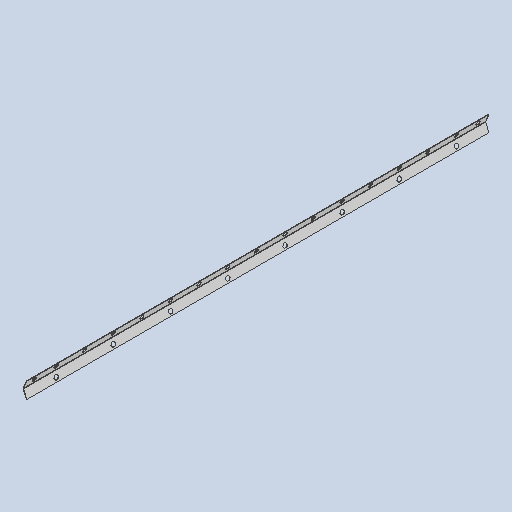
# Autodesk Inventor part: DMF 01 17 опора крышки v2.1
Saved by Autodesk Inventor 2025 (Build 290162010, 162A)
## iProperties
Created: 2024-04-30
Part Number: DMF 01 17 опора крышки v2.1
Material: Generic
Document SubType Name: Sheet Metal
Designer: pokla
Density: 1 g/cm^3
Appearance: Default
Sheet Metal Rule: Default
Flat Pattern Width: 7.47819 cm
Flat Pattern Length: 202 cm
Flat Pattern Area: 1510.6 cm^2
Sheet Metal Width: 74,782 mm
Sheet Metal Length: 2020,000 mm
Sheet Metal Area: 151059,532 mm^2
Stock Number: Барабан_Полка_Крышки
Author: pokla
Autodesk Inventor part; units mm, degrees
ref_plane "YZ Plane" through (0, 0, 0) normal (1, 0, 0) x (0, 1, 0)
ref_plane "XZ Plane" through (0, 0, 0) normal (0, 1, 0) x (-1, 0, 0)
ref_plane "XY Plane" through (0, 0, 0) normal (0, 0, 1) x (1, 0, 0)
sketch "Sketch4" plane through (0, 0, 0) normal (0, 0, 1) x (1, 0, 0)
  line L0 (-195.551234, 195.551234) -> (0, 276.551207) construction
  line L1 (0, 276.551207) -> (195.551234, 195.551234) construction
  line L2 (195.551234, 195.551234) -> (276.551207, 0) construction
  line L3 (276.551207, 0) -> (195.551234, -195.551234) construction
  line L4 (195.551234, -195.551234) -> (0, -276.551207) construction
  line L5 (0, -276.551207) -> (-195.551234, -195.551234) construction
  line L6 (-195.551234, -195.551234) -> (-276.551207, 0) construction
  line L7 (-276.551207, 0) -> (-195.551234, 195.551234) construction
  line L8 (-275.917157, 1.530734) -> (-262.041055, 35.030606)
  line L9 (-275.917157, -1.530734) -> (-262.041055, -35.030606)
  arc A0 (-275.917157, 1.530734) -> (-275.917157, -1.530734) centre (-272.221638, 0) ccw
  point P0 (0, 0)
  point P1 (0, 0)
  point P2 (0, 0)
  dimension "d16" = 511
  dimension "d23" = 36.26
  dimension "d24" = 4
  measures "d16" distance between parallel lines of L7 L3
  measures "d23" distance of L8.start L8.end
  measures "d24" radius of A0
contour flange "Contour Flange1" sketch "Sketch4" thickness 2 bend radius 2 width 2020 along (0, 0, -1) mid plane no both sides no wall seen from (-268.979106, 18.28067, 0) lies toward (0.9238795, -0.3826834, 0) curves L8 A0 L9
bend "Bend2"
corner "Corner2"
sketch "Sketch6" plane through (-275.917157, 1.530734, 0) normal (-0.9238795, 0.3826834, 0) x (0.3826834, 0.9238795, 0)
  circle A0 centre (19.22, 40.75) radius 5.5 construction
  circle A1 centre (19.22, 1979.25) radius 5.5 construction
  line L0 (0, 0) -> (0, 2020)
  line L1 (36.26, 2020) -> (0, 2020)
  line L2 (36.26, 0) -> (0, 0)
  line L3 (27.62, 1974.400258) -> (19.22, 1969.550515)
  line L4 (19.22, 1969.550515) -> (10.82, 1974.400258)
  line L5 (10.82, 1974.400258) -> (10.82, 1984.099742)
  line L6 (10.82, 1984.099742) -> (19.22, 1988.949485)
  line L7 (19.22, 1988.949485) -> (27.62, 1984.099742)
  line L8 (27.62, 1984.099742) -> (27.62, 1974.400258)
  line L9 (27.62, 35.900258) -> (19.22, 31.050515)
  line L10 (19.22, 31.050515) -> (10.82, 35.900258)
  line L11 (10.82, 35.900258) -> (10.82, 45.599742)
  line L12 (10.82, 45.599742) -> (19.22, 50.449485)
  line L13 (19.22, 50.449485) -> (27.62, 45.599742)
  line L14 (27.62, 45.599742) -> (27.62, 35.900258)
  point P0 (104.174711, 0)
  dimension "d36" = 11
  dimension "d41" = 11
  dimension "d93" = 19.22
  dimension "d94" = 40.75
  dimension "d95" = 19.22
  dimension "d96" = 40.75
  dimension "d98" = 16.8
  dimension "d99" = 16.8
  constraints: 24 end point, 2 centre point, 2 coincident, 2 parallel, 26 other
  measures "d36" diameter of A0
  measures "d41" diameter of A1
  measures "d93" distance from line of L0 A0.centre
  measures "d94" distance from line of L2 A0.centre
  measures "d95" distance from line of L0 A1.centre
  measures "d96" distance from line of L1 A1.centre
  measures "d98" distance between parallel lines of L6 L3
  measures "d99" distance between parallel lines of L12 L9
extrude "Extrusion1" cut sketch "Sketch6" against normal up to surface (2 mm away)
sketch "Sketch12" plane through (-275.917157, -1.530734, -2020) normal (-0.9238795, -0.3826834, 0) x (0, 0, 1)
  line L0 (860, -36.26) -> (910, -36.26) construction
  line L1 (910, -36.26) -> (910, -11.26) construction
  line L2 (910, -11.26) -> (860, -11.26) construction
  line L3 (860, -11.26) -> (860, -36.26) construction
  line L4 (2020, 0) -> (0, 0)
  line L5 (889.849742, -12.86) -> (894.699485, -21.26)
  line L6 (894.699485, -21.26) -> (889.849742, -29.66)
  line L7 (889.849742, -29.66) -> (880.150258, -29.66)
  line L8 (880.150258, -29.66) -> (875.300515, -21.26)
  line L9 (875.300515, -21.26) -> (880.150258, -12.86)
  line L10 (880.150258, -12.86) -> (889.849742, -12.86)
  point P0 (2020, -104.174711)
  point P1 (0, -36.26)
  point P2 (1010, 0)
  point P3 (885, -11.26)
  point P4 (885, -21.26)
  point P5 (885, -12.86)
  dimension "d75" = 50
  dimension "d76" = 25
  dimension "d77" = 125
  dimension "magic_d3" = 16.8
  dimension "magic_d2" = 21.26
  constraints: 20 end point, 3 midpoint, 2 parallel, 2 vertical alignment, 1 horizontal, 1 horizontal alignment, 1 perpendicular, 13 other
  measures "d75" distance of L0.start L0.end
  measures "d76" distance of L2.end L0.start
  measures "d77" horizontal distance of point (1010, 0) point (885, -11.26)
  measures "magic_d3" distance between parallel lines of L7 L10
  measures "magic_d2" distance from line of point (885, -21.26) L4
extrude "Extrusion6" cut sketch "Sketch12" against normal through all
mirror "Mirror1" about plane through (0, 0, 0) normal (0, 1, 0) of "Extrusion6"
pattern_linear "Rectangular Pattern4" count 8 spacing 250 along (0, 0, 1) of "Extrusion6", "Mirror1" first direction both ways yes
sketch "Sketch13" plane through (-275.917157, 1.530734, 0) normal (-0.9238795, 0.3826834, 0) x (0.3826834, 0.9238795, 0)
  circle A0 centre (19.22, 1010) radius 5.5 construction
  line L0 (36.26, 0) -> (36.26, 2020)
  line L1 (36.26, 0) -> (0, 0)
  line L2 (27.62, 1005.150258) -> (19.22, 1000.300515)
  line L3 (19.22, 1000.300515) -> (10.82, 1005.150258)
  line L4 (10.82, 1005.150258) -> (10.82, 1014.849742)
  line L5 (10.82, 1014.849742) -> (19.22, 1019.699485)
  line L6 (19.22, 1019.699485) -> (27.62, 1014.849742)
  line L7 (27.62, 1014.849742) -> (27.62, 1005.150258)
  point P0 (104.174711, 0)
  point P1 (36.26, 1010)
  point P2 (35, 910)
  point P3 (35, 1110)
  point P4 (18.13, 0)
  point P5 (27.62, 1010)
  dimension "d83" = 11
  dimension "magic_d1" = 17.04
  dimension "d97" = 16.8
  constraints: 12 end point, 2 horizontal alignment, 2 midpoint, 1 centre point, 1 coincident, 15 other
  measures "d83" diameter of A0
  measures "d97" distance between parallel lines of L4 L7
extrude "Extrusion7" cut sketch "Sketch13" against normal through all
pattern_linear "Rectangular Pattern5" count 7 spacing 250 along (0, 0, 1) of "Extrusion7" first direction both ways yes
equation "\"d77\" = Барабан_Отступ_окна_от_середины"
equation "\"d16\" = Барабан_габарит_по_кассетам - Thickness"
equation "\"d24\" = BendRadius + Thickness"
equation "\"d41\" = d36"
equation "\"d95\" = d93"
equation "\"d96\" = d94"
equation "\"d99\" = d98"
equation "\"d75\" = Барабан_Ширина_окна"
equation "\"d25\" = Thickness"
equation "\"d26\" = BendReliefWidth"
equation "\"d27\" = BendReliefDepth"
equation "\"d28\" = MinimumRemnant"
equation "\"d29\" = TransitionRadius"
equation "\"d30\" = Барабан_длина_листа"
equation "\"d31\" = BendRadius"
equation "\"d33\" = CornerReliefSize"
equation "\"d34\" = GapSize"
equation "\"d35\" = JacobiRadiusSize"
equation "\"BendRadius\" = Thickness"
equation "\"BendReliefWidth\" = Thickness"
equation "\"BendReliefDepth\" = 0.5 * Thickness"
equation "\"CornerReliefSize\" = 4 * Thickness"
equation "\"MinimumRemnant\" = 2 * Thickness"
equation "\"TransitionRadius\" = BendRadius"
equation "\"JacobiRadiusSize\" = BendRadius"
equation "\"GapSize\" = Thickness"
equation "\"Барабан_габарит_по_кассетам\" = 513"
equation "\"Thickness\" = 2"
equation "\"Барабан_Ширина_окна\" = 50"
equation "\"Барабан_длина_листа\" = 2020"
equation "\"Барабан_Отступ_окна_от_середины\" = 125"
body "Solid2"
